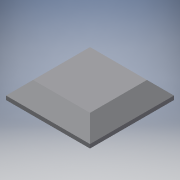
# Autodesk Inventor part: Tripod
Saved by Autodesk Inventor 2016 (Build 200138000, 138)
## iProperties
Created: 2015-08-12
Part Number: Tripod
Material: Generic
Document SubType Name: Modeling
Designer: Kurtis
Density: 1 g/cm^3
Appearance: Default
Author: Kurtis
Autodesk Inventor part; units mm, degrees
ref_plane "YZ Plane" through (0, 0, 0) normal (1, 0, 0) x (0, 1, 0)
ref_plane "XZ Plane" through (0, 0, 0) normal (0, 1, 0) x (-1, 0, 0)
ref_plane "XY Plane" through (0, 0, 0) normal (0, 0, 1) x (1, 0, 0)
sketch "Sketch1" plane through (0, 0, 0) normal (0, 0, 1) x (1, 0, 0)
  line L0 (0, 0) -> (43.5, 0)
  line L1 (43.5, 0) -> (43.5, 43.5)
  line L2 (43.5, 43.5) -> (0, 43.5)
  line L3 (0, 43.5) -> (0, 0)
  dimension "d0" = 43.5
  dimension "d1" = 43.5
  constraints: 8 end point, 2 parallel, 1 horizontal, 1 perpendicular
  measures "d0" distance of L2.end L1.end
  measures "d1" distance of L1.end L0.end
extrude "Extrusion1" add sketch "Sketch1" along normal blind 9
chamfer "Chamfer1" distance 7 angle 45 4 edges at (21.75, 43.5, 9) (0, 21.75, 9) (21.75, 0, 9) (43.5, 21.75, 9)
body "Solid1"
